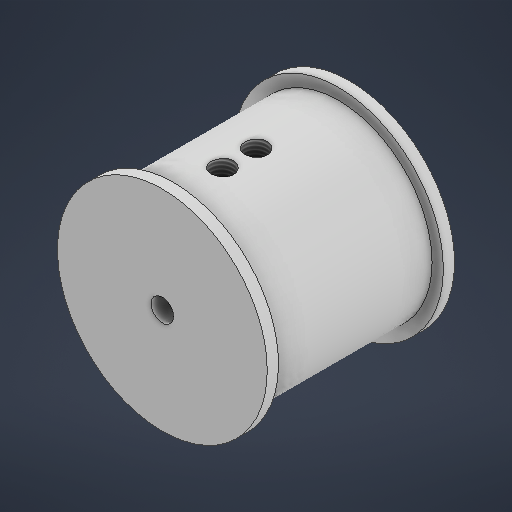
# Autodesk Inventor part: Wheel
Saved by Autodesk Inventor 2026.2 (Build 302298010, 298A)
## iProperties
Created: 2026-03-28
Part Number: Wheel
Material: Všeobecné
Document SubType Name: Modeling
Designer: zak
Density: 1 g/cm^3
Appearance: Výchozí
Author: zak
Autodesk Inventor part; units mm, degrees
ref_plane "YZ Plane" through (0, 0, 0) normal (1, 0, 0) x (0, 1, 0)
ref_plane "XZ Plane" through (0, 0, 0) normal (0, 1, 0) x (-1, 0, 0)
ref_plane "XY Plane" through (0, 0, 0) normal (0, 0, 1) x (1, 0, 0)
sketch "Náčrt1" plane through (0, 0, 0) normal (0, 0, 1) x (1, 0, 0)
  circle A0 centre (0, 0) radius 14
  dimension "d0" = 28
  constraints: 1 centre point, 1 coincident
  measures "d0" diameter of A0
extrude "Vysunutí1" add sketch "Náčrt1" along normal mid plane 25
sketch "Náčrt2" plane through (0, 0, 0) normal (1, 0, 0) x (0, 1, 0)
  line L0 (-14, -12.5) -> (14, -12.5) projected
  line L1 (14, 12.5) -> (-14, 12.5) projected
  line L2 (14, -12.5) -> (14, 12.5) projected
  line L3 (14, 11) -> (12.5, 11)
  line L4 (12.5, 11) -> (12.5, -11)
  line L5 (12.5, -11) -> (14, -11)
  line L6 (14, -11) -> (14, 11)
  line L7 (14, 0) -> (-14, 0) construction
  line L8 (-14, -12.5) -> (-14, 12.5) projected
  line L9 (0, 12.5) -> (0, -12.5) construction
  point P0 (0, 0)
  point P1 (14, -11)
  dimension "d4" = 11
  dimension "d5" = 12.5
  constraints: 12 end point, 4 midpoint, 2 parallel, 1 horizontal, 1 perpendicular, 1 point on line, 1 other
  measures "d4" distance between parallel lines of L7 L3
  measures "d5" distance between parallel lines of L9 L4
revolve "Rotace1" cut sketch "Náčrt2" angle 360 about axis through (0, 0, 12.5) along (0, 0, -1) contours L5 L4 L3 L2
sketch "Náčrt3" plane through (0, 0, -12.5) normal (0, 0, -1) x (-1, 0, 0)
  line L0 (-6, 5) -> (6, 5)
  line L1 (6, 5) -> (6, -5)
  line L2 (6, -5) -> (-6, -5)
  line L3 (-6, -5) -> (-6, 5)
  line L4 (-6, 5) -> (6, -5) construction
  line L5 (6, 5) -> (-6, -5) construction
  circle A0 centre (0, 0) radius 9
  dimension "d7" = 12
  dimension "d8" = 10
  dimension "d9" = 18
  constraints: 12 end point, 2 midpoint, 2 parallel, 1 centre point, 1 coincident, 1 horizontal, 1 perpendicular
  measures "d7" distance of L1.end L2.end
  measures "d8" distance of L0.end L1.end
  measures "d9" diameter of A0
hole "Díra1" at (0, 0, -12.5) direction (0, 0, 1) diameter 18 depth 10
sketch "Náčrt4" plane through (0, 0, 12.5) normal (0, 0, 1) x (1, 0, 0)
  circle A0 centre (0, 0) radius 14 projected
  constraints: 1 coincident
hole "Díra2" at (0, 0, 12.5) direction (0, 0, -1) diameter 3 end through all
ref_plane "Pracovní rovina1" through (0, 12.5, 0) normal (0, -1, 0) x (1, 0, 0)
sketch "Náčrt5" plane through (0, 12.5, 0) normal (0, -1, 0) x (1, 0, 0)
  line L0 (1.5, -2.5) -> (-1.5, -2.5) projected
  line L1 (-9, -2.5) -> (9, -2.5) projected
  line L2 (0, 0) -> (0, -10.7479) construction
  point P0 (0, 4.5)
  dimension "d24" = 2.5
  dimension "d25" = 4.5
  constraints: 2 end point, 2 point on line, 1 vertical
  measures "d24" distance from line of L1 point (0, 0)
  measures "d25" distance of point (0, 0) point (0, 4.5)
hole "Díra3" at (0, 12.5, 0) at (0, 12.5, 4.5) direction (0, -1, 0) diameter 3 depth 12.5
thread "Závit1" size "M3x0.5" class "6H" standard "ISO Metric profile" full length
thread "Závit2" size "M3x0.5" class "6H" standard "ISO Metric profile" full length
chamfer "Zkosení1" distance 1 angle 45 1 edges at (0, -9, -12.5)
fillet "Zaoblení1" radius 1 1 edges at (0, -9, -2.5)
